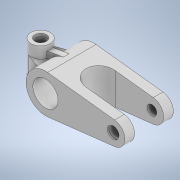
# Autodesk Inventor part: Rubia_ASR3
Saved by Autodesk Inventor 2021 (Build 250183000, 183)
## iProperties
Created: 2021-03-25
Part Number: Rubia_ASR3
Material: Genérico
Document SubType Name: Modeling
Designer: rubia
Density: 1 g/cm^3
Appearance: Padrão
Author: rubia
Autodesk Inventor part; units mm, degrees
ref_plane "YZ Plane" through (0, 0, 0) normal (1, 0, 0) x (0, 1, 0)
sketch "Esboço1" plane through (0, 0, 0) normal (0, 0, 1) x (1, 0, 0)
  arc A0 (5.7143, 49.6724) -> (5.7143, -49.6724) centre (0, 0) ccw
  arc A1 (178.4286, -29.8034) -> (178.4286, 29.8034) centre (175, 0) ccw
  line L0 (5.7143, 49.6724) -> (178.4286, 29.8034)
  line L1 (0, 0) -> (175, 0) construction
  line L2 (5.7143, -49.6724) -> (178.4286, -29.8034)
  circle A2 centre (0, 0) radius 32.5
  circle A3 centre (175, 0) radius 12.5
  point P0 (-54.0476, 56.5474)
  point P1 (215.9085, 25.4918)
  point P2 (-54.0476, -56.5474)
  point P3 (215.9085, -25.4918)
  dimension "d0" = 100
  dimension "d1" = 60
  dimension "d2" = 175
  dimension "d3" = 65
  dimension "d4" = 25
  constraints: 6 end point, 4 centre point, 4 point on circle, 3 coincident, 2 symmetric about line, 2 tangent, 1 horizontal, 1 horizontal alignment
  measures "d0" diameter of A0
  measures "d1" diameter of A1
  measures "d2" distance of L1.end point (0, 0)
  measures "d3" diameter of A2
  measures "d4" diameter of A3
extrude "Extrusão1" add sketch "Esboço1" along normal blind 125
ref_plane "Plano de trabalho1" through (0, -25, 0) normal (0, 1, 0) x (-1, 0, 0)
sketch "Esboço2" plane through (0, -25, 0) normal (0, 1, 0) x (-1, 0, 0)
  line L0 (0, 0) -> (0, 125) construction
  line L1 (50, 125) -> (-5.7143, 125) construction
  line L2 (0, 62.5) -> (109.1848, 62.5) construction
  circle A0 centre (75, 62.5) radius 25
  dimension "d8" = 50
  dimension "d9" = 75
  constraints: 4 end point, 2 point on line, 1 centre point, 1 horizontal, 1 midpoint, 1 vertical
  measures "d8" diameter of A0
  measures "d9" distance from line of L0 A0.centre
extrude "Extrusão2" add sketch "Esboço2" along normal blind 80
sketch "Esboço3" plane through (0, -25, 0) normal (0, 1, 0) x (-1, 0, 0)
  circle A0 centre (75, 62.5) radius 25 projected
  arc A1 (83.5505, 85.9923) -> (83.5505, 39.0077) centre (75, 62.5) ccw
  line L0 (83.5505, 39.0077) -> (39.6496, 23.0291)
  line L1 (50, 125) -> (-5.7143, 125) projected
  line L2 (75, 62.5) -> (-32.0182, 62.5) construction
  line L3 (83.5505, 85.9923) -> (39.6496, 101.9709)
  line L4 (39.6496, 23.0291) -> (39.6496, 101.9709)
  point P0 (0, 0)
  point P1 (94.387, 42.9518)
  point P2 (9.9213, 12.2089)
  point P3 (94.387, 82.0482)
  point P4 (9.9213, 112.7911)
  point P5 (83.5505, 39.0077)
  dimension "d12" = 20
  constraints: 8 end point, 2 point on circle, 2 symmetric about line, 1 centre point, 1 coincident, 1 horizontal, 1 tangent, 1 vertical
  measures "d12" angle of L1 L0
extrude "Extrusão3" add sketch "Esboço3" along normal blind 50 contours A0 L0 L4 L3
ref_plane "Plano de trabalho2" through (0, 0, 62.5) normal (0, 0, 1) x (1, 0, 0)
sketch "Esboço4" plane through (0, 0, 62.5) normal (0, 0, 1) x (1, 0, 0)
  line L0 (-50, 55) -> (-100, 55) projected
  line L1 (-75, 37.5468) -> (-75, 0)
  arc A0 (-8.6824, 49.2404) -> (-50, 0) centre (0, 0) ccw
  line L2 (-75, 0) -> (-50, 0)
  line L3 (-75, 37.5468) -> (-8.6824, 49.2404)
  dimension "d16" = 100
  dimension "d17" = 80
  constraints: 6 end point, 2 point on circle, 1 centre point, 1 coincident, 1 horizontal, 1 tangent, 1 vertical
  measures "d16" diameter of A0
  measures "d17" angle of L3 L1
extrude "Extrusão4" add sketch "Esboço4" along normal mid plane 15
sketch "Esboço5" plane through (0, 0, 0) normal (0, 1, 0) x (-1, 0, 0)
  line L0 (0, 0) -> (0, 125) construction
  line L1 (0, 62.5) -> (-205, 62.5) construction
  line L2 (-205, 0) -> (-205, 125) construction
  arc A0 (-80, 25) -> (-80, 100) centre (-80, 62.5) ccw
  line L3 (-80, 25) -> (-214.9719, 25)
  line L4 (-80, 100) -> (-214.9719, 100)
  line L5 (-214.9719, 100) -> (-214.9719, 25)
  dimension "d20" = 75
  dimension "d21" = 80
  constraints: 10 end point, 2 horizontal, 2 midpoint, 2 point on circle, 1 centre point, 1 perpendicular, 1 point on line, 1 tangent, 1 vertical
  measures "d20" diameter of A0
  measures "d21" distance of A0.centre L1.start
extrude "Extrusão5" cut sketch "Esboço5" against normal through all both and the other way through all
sketch "Esboço6" plane through (-75, 55, 62.5) normal (0, 1, 0) x (1, 0, 0)
  point P0 (75, 62.5)
  point P1 (0, 0)
  point P2 (0, 0)
  constraints: 1 coincident
hole "Furo1" at (-75, 55, 62.5) at (-75, 55, 62.5) direction (0, -1, 0) diameter 25 end through all counterbore diameter 30 counterbore depth 8
sketch "Esboço7" plane through (0, 0, 125) normal (0, 0, 1) x (1, 0, 0)
  circle A0 centre (175, 0) radius 12.5 projected
  circle A1 centre (175, 0) radius 15
  point P0 (0, 0)
  dimension "d31" = 30
  constraints: 1 centre point, 1 coincident
  measures "d31" diameter of A1
extrude "Extrusão6" cut sketch "Esboço7" against normal blind 2.5
sketch "Esboço8" plane through (0, 0, 0) normal (0, 0, -1) x (-1, 0, 0)
  circle A0 centre (-175, 0) radius 12.5 projected
  circle A1 centre (-175, 0) radius 15
  point P0 (0, 0)
  dimension "d34" = 30
  constraints: 1 centre point, 1 coincident
  measures "d34" diameter of A1
extrude "Extrusão7" cut sketch "Esboço8" against normal blind 2.5
